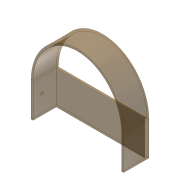
# Autodesk Inventor part: Bucket Flap
Saved by Autodesk Inventor 2015 SP1 (Build 190203100, 203)
## iProperties
Created: 2015-01-24
Part Number: Bucket Flap
Material: Polycarbonate, Clear
Document SubType Name: Modeling
Designer: rihoobler
Density: 1.2 g/cm^3
Appearance: Polycarbonate - Smoked
Author: rihoobler
Autodesk Inventor part; units mm, degrees
ref_plane "YZ Plane" through (0, 0, 0) normal (1, 0, 0) x (0, 1, 0)
ref_plane "XZ Plane" through (0, 0, 0) normal (0, 1, 0) x (-1, 0, 0)
sketch "Sketch1" plane through (0, 0, 0) normal (0, 0, 1) x (1, 0, 0)
  line L0 (139.7, 0) -> (139.7, 50.8)
  line L1 (0, 50.8) -> (0, 0)
  ellipse E0 centre (69.85, 50.8) end of major axis (139.7, 50.8) minor radius 76.2 (139.7, 50.8) -> (0, 50.8) ccw
  line L2 (136.525, 50.8) -> (136.525, 3.175)
  line L3 (3.175, 3.175) -> (3.175, 50.8)
  line L4 (3.175, 3.175) -> (3.175, 0)
  line L5 (136.525, 3.175) -> (136.525, 0)
  line L6 (0, 0) -> (3.175, 0)
  line L7 (136.525, 0) -> (139.7, 0)
  spline S0 degree 5 poles (3.175, 50.8) (3.175, 52.444) (3.2172, 54.088) (3.3017, 55.7305) (4.0773, 65.7654) (6.4328, 75.6371) (9.4981, 83.5865) (17.5722, 98.0931) (29.3701, 109.7459) (35.928, 114.5559) (50.1357, 121.8737) (65.8938, 124.4523) (73.8062, 124.4523) (89.5643, 121.8737) (103.772, 114.5559) (110.3299, 109.7459) (122.1278, 98.0931) (130.2019, 83.5865) (133.2672, 75.6371) (135.6227, 65.7654) (136.3983, 55.7305) (136.4828, 54.088) (136.525, 52.444) (136.525, 50.8) knots 0 0 0 0 0 0 0.03744 0.03744 0.03744 0.22914 0.22914 0.22914 0.411521 0.411521 0.411521 0.588479 0.588479 0.588479 0.77086 0.77086 0.77086 0.96256 0.96256 0.96256 1 1 1 1 1 1
  dimension "d0" = 139.7
  dimension "d1" = 50.8
  constraints: 16 end point, 6 perpendicular, 3 parallel, 2 horizontal, 1 horizontal alignment, 6 other
  measures "d0" distance of L1.start L0.end
  measures "d1" distance of L0.end L0.start
extrude "Extrusion1" add sketch "Sketch1" along normal blind 38.1
ref_plane "Work Plane1" through (136.525, 0, 0) normal (0, -1, 0) x (1, 0, 0)
sketch "Sketch2" plane through (136.525, 0, 0) normal (0, -1, 0) x (1, 0, 0)
  line L0 (-136.525, 0) -> (3.175, 0)
  line L1 (3.175, 0) -> (3.175, 3.175)
  line L2 (3.175, 3.175) -> (-136.525, 3.175)
  line L3 (-136.525, 3.175) -> (-136.525, 0)
  dimension "d7" = 139.7
  dimension "d8" = 3.175
  constraints: 8 end point, 2 parallel, 1 horizontal, 1 perpendicular
  measures "d7" distance of L2.end L1.end
  measures "d8" distance of L1.end L0.end
extrude "Extrusion2" add sketch "Sketch2" against normal blind 50.8
sketch "Sketch3" plane through (0, 0, 38.1) normal (-1, 0, 0) x (0, 0, 1)
  circle A0 centre (-15.138, 26.5498) radius 1.85
  point P0 (-38.1, 0)
  dimension "d11" = 3.7
  constraints: 1 centre point, 1 coincident
  measures "d11" diameter of A0
extrude "Extrusion3" cut sketch "Sketch3" against normal blind 50.8
body "Solid1"
